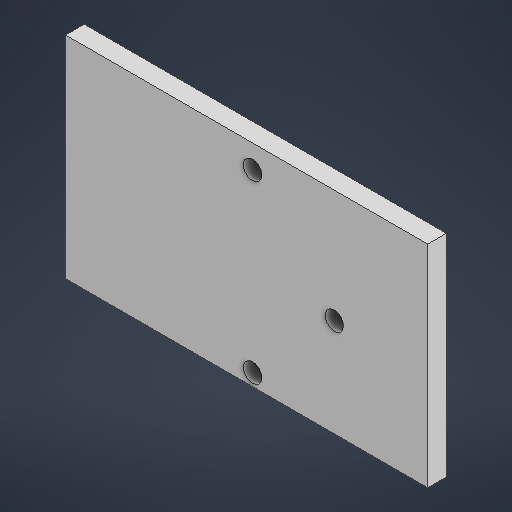
# Autodesk Inventor part: крышка захвата
Saved by Autodesk Inventor 2025 (Build 290162000, 162)
## iProperties
Created: 2025-02-22
Part Number: крышка захвата
Material: Типовые
Document SubType Name: Modeling
Designer: Phantom
Density: 1 g/cm^3
Appearance: По умолчанию
Author: Phantom
Autodesk Inventor part; units mm, degrees
ref_plane "YZ Plane" through (0, 0, 0) normal (1, 0, 0) x (0, 1, 0)
ref_plane "XZ Plane" through (0, 0, 0) normal (0, 1, 0) x (-1, 0, 0)
ref_plane "XY Plane" through (0, 0, 0) normal (0, 0, 1) x (1, 0, 0)
sketch "Эскиз1" plane through (0, 0, 0) normal (0, 0, 1) x (1, 0, 0)
  circle A0 centre (-2.4533, -5.5681) radius 1.6
  line L0 (27.5467, -7.6681) -> (1.5467, -7.6681)
  line L1 (-6.4533, -7.6681) -> (-34.4903, -7.6681)
  line L2 (-34.4903, -7.6681) -> (-6.4533, -7.6681)
  line L3 (1.5467, -7.6681) -> (27.5467, -7.6681)
  line L4 (27.5467, -7.6681) -> (27.5467, 28.4819)
  line L5 (27.5467, 28.4819) -> (-2.4533, 28.4819)
  line L6 (-2.4533, 28.4819) -> (-34.4903, 28.4819)
  line L7 (-34.4903, 28.4819) -> (-34.4903, -7.6681)
  line L8 (-34.4903, 13.2319) -> (-34.4903, 5.0319)
  line L9 (-34.4903, 3.2319) -> (-34.4903, -7.6681)
  circle A1 centre (11.5467, 9.1319) radius 1.575
  circle A2 centre (-2.4533, 24.4819) radius 1.6
  line L10 (-6.4533, -7.6681) -> (1.5467, -7.6681)
  point P0 (0, 0)
  point P1 (-2.4533, -2.0181)
  point P2 (1.5467, -7.6681)
  constraints: 22 end point, 3 centre point, 1 horizontal
extrude "Выдавливание1" add sketch "Эскиз1" along normal blind 3.2
